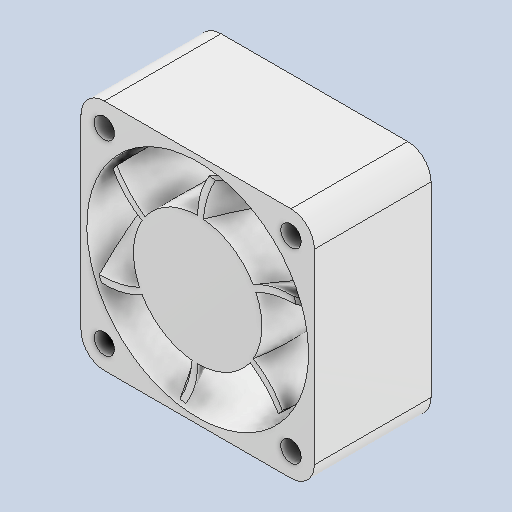
# Autodesk Inventor part: 4020 AXIAL FAN
Saved by Autodesk Inventor 2022 (Build 260153070, 153G)
## iProperties
Created: 2022-01-01
Part Number: 4020 AXIAL FAN
Material: ABS Plastic
Document SubType Name: Modeling
Designer: a laptop
Density: 1.06 g/cm^3
Appearance: Smooth - White
Author: a laptop
Autodesk Inventor part; units mm, degrees
ref_plane "YZ Plane" through (0, 0, 0) normal (1, 0, 0) x (0, 1, 0)
ref_plane "XZ Plane" through (0, 0, 0) normal (0, 1, 0) x (-1, 0, 0)
sketch "Sketch1" plane through (0, 0, 0) normal (0, 0, 1) x (1, 0, 0)
  line L0 (-16, 20) -> (16, 20)
  line L1 (20, 16) -> (20, -16)
  line L2 (16, -20) -> (-16, -20)
  line L3 (-20, -16) -> (-20, 16)
  arc A0 (-16, 20) -> (-20, 16) centre (-16, 16) ccw
  arc A1 (20, 16) -> (16, 20) centre (16, 16) ccw
  arc A2 (16, -20) -> (20, -16) centre (16, -16) ccw
  arc A3 (-20, -16) -> (-16, -20) centre (-16, -16) ccw
  circle A4 centre (-16, 16) radius 1.75
  circle A5 centre (16, -16) radius 1.75
  circle A6 centre (16, 16) radius 1.75
  circle A7 centre (-16, -16) radius 1.75
  circle A8 centre (0, 0) radius 19
  line L4 (-20, 0) -> (20, 0) construction
  line L5 (0, 20) -> (0, -20) construction
  point P0 (-20, 20)
  point P1 (20, 20)
  dimension "d0" = 40
  dimension "d3" = 32
  dimension "d4" = 3.5
  dimension "d5" = 3.5
  dimension "d6" = 3.5
  dimension "d7" = 3.5
  dimension "d8" = 38
  constraints: 12 end point, 9 centre point, 8 point on circle, 8 tangent, 6 coincident, 6 midpoint, 4 point on line, 3 equal radius, 3 perpendicular, 2 parallel, 1 horizontal
  measures "d0" distance of point (-20, 20) point (20, 20)
  measures "d3" distance of A1.centre A0.centre
  measures "d4" diameter of A4
  measures "d5" diameter of A5
  measures "d6" diameter of A6
  measures "d7" diameter of A7
  measures "d8" diameter of A8
extrude "Extrusion1" add sketch "Sketch1" along normal blind 20
sketch "Sketch2" plane through (0, 0, 20) normal (0, 0, 1) x (1, 0, 0)
  circle A0 centre (0, 0) radius 11
  dimension "d11" = 22
  constraints: 1 centre point, 1 coincident
  measures "d11" diameter of A0
extrude "Extrusion2" add sketch "Sketch2" against normal blind 18
fillet "Fillet1" radius 2 1 edges at (-11, 0, 2)
sketch "Sketch3" plane through (0, 0, 20) normal (0, 0, 1) x (1, 0, 0)
  circle A0 centre (0, 0) radius 11
  arc A1 (3.590901, 18.657584) -> (0.958713, 10.958142) centre (17.861274, 9.479359) ccw
  arc A2 (2.644289, 18.815093) -> (0, 11) centre (12.870747, 11) ccw
  circle A3 centre (0, 0) radius 19
  line L0 (0, 11) -> (0, 0) construction
  line L1 (0, 0) -> (0.958713, 10.958142) construction
  line L2 (2.644289, 18.815093) -> (3.590901, 18.657584) construction
  line L3 (0, 11) -> (0.958713, 10.958142) construction
  line L4 (2.644289, 18.815093) -> (0, 0) construction
  dimension "d15" = 38
  dimension "d17" = 5
  dimension "d19" = 8
  constraints: 10 end point, 8 point on circle, 3 centre point, 2 tangent, 1 coincident, 1 equal length, 1 vertical alignment
  measures "d15" diameter of A3
  measures "d17" angle of L1 L0
  measures "d19" angle of L4 L0
ref_plane "Work Plane1" through (0, 0, 4) normal (0, 0, 1) x (1, 0, 0)
sketch "Sketch4" plane through (0, 0, 4) normal (0, 0, 1) x (1, 0, 0)
  circle A0 centre (0, 0) radius 19
  arc A1 (11.697568, 14.972204) -> (5.5, 9.526279) centre (16.646394, 3.090906) ccw
  arc A2 (12.438603, 14.362491) -> (6.309341, 9.010672) centre (20.207997, -0.721271) ccw
  line L0 (6.309341, 9.010672) -> (0, 0) construction
  line L1 (0, 0) -> (5.5, 9.526279) construction
  line L2 (12.438603, 14.362491) -> (11.697568, 14.972204) construction
  line L3 (6.309341, 9.010672) -> (5.5, 9.526279) construction
  line L4 (11.697568, 14.972204) -> (0, 0) construction
  line L5 (0, 0) -> (0, 11) construction
  circle A3 centre (0, 0) radius 11
  dimension "d21" = 5
  dimension "d23" = 8
  dimension "d24" = 30
  constraints: 12 end point, 8 point on circle, 3 coincident, 2 centre point, 2 tangent, 1 equal length, 1 vertical
  measures "d21" angle of L1 L0
  measures "d23" angle of L1 L4
  measures "d24" angle of L5 L1
sketch "Sketch3 outline for Loft2" plane through (0, 0, 20) normal (0, 0, 1) x (1, 0, 0)
  arc A0 (0.958713, 10.958142) -> (3.590901, 18.657584) centre (17.861274, 9.479359) cw
  arc A1 (0, 11) -> (0.958713, 10.958142) centre (0, 0) cw
  arc A2 (2.644289, 18.815093) -> (0, 11) centre (12.870747, 11) ccw
  arc A3 (3.590901, 18.657584) -> (2.644289, 18.815093) centre (0, 0) ccw
sketch "Sketch4 outline for Loft2" plane through (0, 0, 4) normal (0, 0, 1) x (1, 0, 0)
  arc A0 (12.438603, 14.362491) -> (11.697568, 14.972204) centre (0, 0) ccw
  arc A1 (6.309341, 9.010672) -> (12.438603, 14.362491) centre (20.207997, -0.721271) cw
  arc A2 (5.5, 9.526279) -> (6.309341, 9.010672) centre (0, 0) cw
  arc A3 (11.697568, 14.972204) -> (5.5, 9.526279) centre (16.646394, 3.090906) ccw
loft "Loft2" add profiles "Sketch3 outline for Loft2", "Sketch4 outline for Loft2"
pattern_circular "Circular Pattern1" count 6 over 360 about axis through (0, 0, 4) along (0, 0, -1) of "Loft2"
sketch "Sketch5" plane through (0, 0, 2) normal (0, 0, -1) x (-1, 0, 0)
  circle A0 centre (0, 0) radius 19 projected
  circle A1 centre (0, 0) radius 18
  dimension "d36" = 1
  constraints: 1 centre point, 1 coincident
  measures "d36" radial gap between concentric circles of A0 A1
extrude "Extrusion3" cut sketch "Sketch5" against normal blind 18
body "Solid1"
